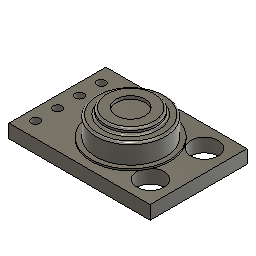
wearable+infrared+thermometer+ring+v1 (Autodesk Fusion 360 archive; units mm, degrees)
design "GY-906 X"
Autodesk Fusion 360 part; units mm, degrees
sketch "Sketch1" plane through (0, 0, 0) normal (0, 1, 0) x (1, 0, 0)
  line L0 (-8.9546, -5.9752) -> (7.6454, -5.9752)
  line L1 (7.6454, -5.9752) -> (7.6454, 5.4248)
  line L2 (7.6454, 5.4248) -> (-8.9546, 5.4248)
  line L3 (-8.9546, 5.4248) -> (-8.9546, -5.9752)
  circle A0 centre (-7.6106, 3.5462) radius 0.5
  circle A1 centre (-7.6106, 0.9716) radius 0.5
  circle A2 centre (-7.6106, -1.6031) radius 0.5
  circle A3 centre (-7.6106, -4.1778) radius 0.5
  circle A4 centre (-0.1943, -0.421) radius 4.615
  circle A5 centre (-0.1943, -0.421) radius 4.075
  circle A6 centre (-0.1943, -0.421) radius 3
  circle A7 centre (-0.1943, -0.421) radius 1.7
  circle A8 centre (5.1007, 2.9633) radius 1.6
  circle A9 centre (5.1007, -3.3843) radius 1.6
  dimension "d1" = 16.6
  dimension "d2" = 11.4
  dimension "d3" = 1
  dimension "d6" = 0
  dimension "d7" = -7.724
  dimension "d8" = 9.23
  dimension "d9" = 8.15
  dimension "d10" = 6
  dimension "d11" = 3.4
  dimension "d12" = 3.2
  dimension "d13" = 3.2
  constraint horizontal L0
  constraint vertical L1
  constraint horizontal L2
  constraint vertical L3
  constraint concentric A4 A5
  constraint concentric A4 A6
  constraint concentric A4 A7
  measures "d1" distance of L0.start L0.end
  measures "d2" distance of L0.start L2.end
  measures "d3" diameter of A0
  measures "d8" diameter of A4
  measures "d9" diameter of A5
  measures "d10" diameter of A6
  measures "d11" diameter of A7
  measures "d12" diameter of A8
  measures "d13" diameter of A9
extrude "Extrude1" add sketch "Sketch1" against normal blind 1.6 contours L0 L1 L2 L3 | A4 A9 | A5 | A6 | A7 picked at (3.1257, -3.3478)
extrude "Extrude2" add sketch "Sketch1" along normal blind 0.2 contours A4 A9 | A4 A9 picked at (3.1257, -3.3478) picked at (3.7696, -2.6849)
extrude "Extrude3" add sketch "Sketch1" along normal blind 2.5 contours A5
extrude "Extrude4" add sketch "Sketch1" along normal blind 3.2 contours A6
extrude "Extrude5" add sketch "Sketch1" along normal blind 2.839 contours A7
fillet "Fillet1" radius 0.23 3 edges at (-2.9913, 3.2, 1.5059) (-2.9913, 2.5, -0.6638) (-3.9935, 2.5, 1.8946)
